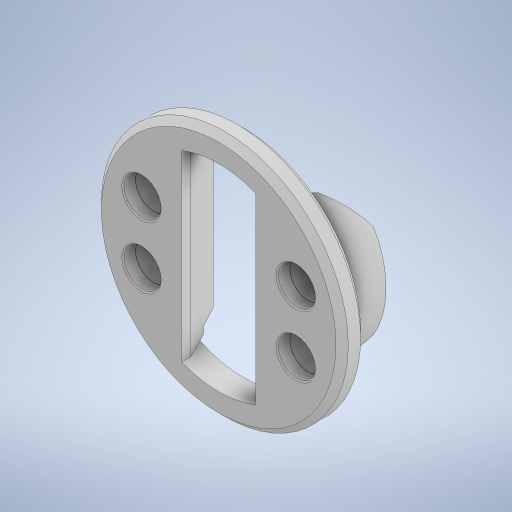
# Autodesk Inventor part: arm_head
Saved by Autodesk Inventor 2023.4 (Build 274418000, 418)
## iProperties
Created: 2024-02-15
Part Number: arm_head
Material: Generic
Document SubType Name: Modeling
Designer: aaron
Density: 1 g/cm^3
Appearance: Default
Author: aaron
Autodesk Inventor part; units mm, degrees
ref_plane "YZ Plane" through (0, 0, 0) normal (1, 0, 0) x (0, 1, 0)
ref_plane "XZ Plane" through (0, 0, 0) normal (0, 1, 0) x (-1, 0, 0)
ref_plane "XY Plane" through (0, 0, 0) normal (0, 0, 1) x (1, 0, 0)
sketch "Sketch1" plane through (0, 0, 0) normal (0, 0, 1) x (1, 0, 0)
  circle A0 centre (0, 0) radius 15.025
  dimension "d0" = 30.05
  constraints: 1 centre point, 1 coincident
  measures "d0" diameter of A0
extrude "Extrusion1" add sketch "Sketch1" along normal blind 7.1
sketch "Sketch2" plane through (0, 0, 7.1) normal (0, 0, 1) x (1, 0, 0)
  circle A0 centre (0, 0) radius 16
  dimension "d3" = 32
  constraints: 1 centre point, 1 coincident
  measures "d3" diameter of A0
extrude "Extrusion2" add sketch "Sketch2" along normal blind 1
sketch "Sketch3" plane through (0, 0, 8.1) normal (0, 0, 1) x (1, 0, 0)
  circle A0 centre (0, 0) radius 20
  dimension "d6" = 40
  constraints: 1 centre point, 1 coincident
  measures "d6" diameter of A0
extrude "Extrusion3" add sketch "Sketch3" along normal blind 4
sketch "Sketch4" plane through (0, 0, 0) normal (0, 0, -1) x (-1, 0, 0)
  circle A0 centre (0, 0) radius 16 projected
  line L0 (6, 25.2369) -> (-6, 25.2369)
  line L1 (-6, 25.2369) -> (-6, -24.7248)
  line L2 (-6, -24.7248) -> (6, -24.7248)
  line L3 (6, -24.7248) -> (6, 25.2369)
  point P0 (6, -14.8324)
  point P1 (6, 14.8324)
  point P2 (-6, 14.8324)
  point P3 (-6, -14.8324)
  dimension "d9" = 6
  dimension "d10" = 6
  constraints: 8 end point, 2 parallel, 1 horizontal, 1 perpendicular
  measures "d9" distance from line of L1 point (0, 0)
  measures "d10" distance from line of L3 point (0, 0)
extrude "Extrusion4" cut sketch "Sketch4" against normal through all contours L3 A0 L1
chamfer "Chamfer1" distance 7 angle 45 2 edges at (-6, 0, 0) (6, 0, 0)
chamfer "Chamfer3" distance 1 angle 45 2 edges at (-20, 0, 8.1) (-20, 0, 12.1)
sketch "Sketch6" plane through (0, 0, 12.1) normal (0, 0, 1) x (1, 0, 0)
  circle A0 centre (-12.5, -5) radius 1.55
  arc A1 (-13, 7.5333) -> (-13, -7.5333) centre (0, 0) ccw projected
  line L0 (-13, -7.5333) -> (-13, 7.5333) projected
  line L1 (0, 0) -> (0, -4.0369)
  line L2 (0, 0) -> (-1.7679, 0)
  circle A2 centre (12.5, -5) radius 1.55
  circle A3 centre (-12.5, 5) radius 1.55
  circle A4 centre (12.5, 5) radius 1.55
  dimension "d22" = 5
  dimension "d23" = 12.5
  dimension "d24" = 3.1
  constraints: 4 centre point, 4 end point, 3 symmetric about line, 1 horizontal, 1 vertical, 3 other
  measures "d22" vertical distance of A0.centre point (0, 0)
  measures "d23" horizontal distance of point (0, 0) A0.centre
  measures "d24" diameter of A0
extrude "Extrusion5" cut sketch "Sketch6" against normal through all contours A0 L0 | L0 A0 | A3 L0 | L0 A3 | A2 | A4
sketch "Sketch7" plane through (0, 0, 12.1) normal (0, 0, 1) x (1, 0, 0)
  circle A0 centre (-12.5, -5) radius 1.55 projected
  circle A1 centre (-12.5, 5) radius 1.55 projected
  circle A2 centre (12.5, 5) radius 1.55 projected
  circle A3 centre (12.5, -5) radius 1.55 projected
  circle A4 centre (-12.5, -5) radius 3
  circle A5 centre (-12.5, 5) radius 3
  circle A6 centre (12.5, 5) radius 3
  circle A7 centre (12.5, -5) radius 3
  point P0 (0, 0)
  dimension "d27" = 6
  dimension "d28" = 6
  dimension "d29" = 6
  dimension "d30" = 6
  constraints: 4 centre point, 4 coincident
  measures "d27" diameter of A4
  measures "d28" diameter of A7
  measures "d29" diameter of A6
  measures "d30" diameter of A5
extrude "Extrusion6" cut sketch "Sketch7" against normal blind 2
chamfer "Chamfer4" distance 1.4 angle 45 4 edges at (-14.05, -5, 10.1) (-14.05, 5, 10.1) (10.95, 5, 10.1) (10.95, -5, 10.1)
chamfer "Chamfer5" distance 0.2 angle 45 4 edges at (-15.5, -5, 12.1) (-15.5, 5, 12.1) (9.5, -5, 12.1) (9.5, 5, 12.1)
chamfer "Chamfer8" distance 3.6 angle 45 2 edges at (-6, 0, 7) (6, 0, 7)
equation "\"d9\" = d10"
equation "\"d28\" = d27"
equation "\"d29\" = d27"
equation "\"d30\" = d27"
body "Solid1"
